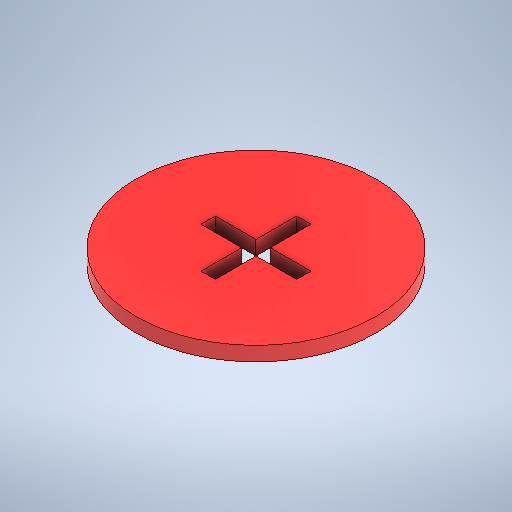
# Autodesk Inventor part: Base Arvore
Saved by Autodesk Inventor 2025 (Build 290162000, 162)
## iProperties
Created: 2024-12-03
Part Number: Base Arvore
Material: Generic
Document SubType Name: Modeling
Designer: Inteli
Density: 1 g/cm^3
Appearance: Light Red
Author: Inteli
Autodesk Inventor part; units mm, degrees
ref_plane "YZ Plane" through (0, 0, 0) normal (1, 0, 0) x (0, 1, 0)
ref_plane "XZ Plane" through (0, 0, 0) normal (0, 1, 0) x (-1, 0, 0)
ref_plane "XY Plane" through (0, 0, 0) normal (0, 0, 1) x (1, 0, 0)
sketch "Sketch1" plane through (0, 0, 0) normal (0, 1, 0) x (-1, 0, 0)
  circle A0 centre (0, 0) radius 25
  line L0 (10, 1.5) -> (-10, 1.5)
  line L1 (-10, 1.5) -> (-10, -1.5)
  line L2 (-10, -1.5) -> (10, -1.5)
  line L3 (10, -1.5) -> (10, 1.5)
  line L4 (1.5, 10) -> (-1.5, 10)
  line L5 (-1.5, 10) -> (-1.5, -10)
  line L6 (-1.5, -10) -> (1.5, -10)
  line L7 (1.5, -10) -> (1.5, 10)
  point P0 (-1.5, 1.5)
  point P1 (1.5, 1.5)
  point P2 (1.5, -1.5)
  point P3 (-1.5, -1.5)
  dimension "d0" = 50
  dimension "d1" = 20
  dimension "d2" = 3
  dimension "d3" = 1.5
  dimension "d4" = 10
  dimension "d5" = 3
  dimension "d6" = 20
  dimension "d7" = 10
  dimension "d8" = 1.5
  constraints: 16 end point, 4 parallel, 2 horizontal, 2 perpendicular, 1 centre point, 1 coincident
  measures "d0" diameter of A0
  measures "d1" distance of L2.end L1.end
  measures "d2" distance of L1.end L0.end
  measures "d3" distance from line of L2 point (0, 0)
  measures "d4" distance from line of point (0, 0) L3
  measures "d5" distance of L6.end L5.end
  measures "d6" distance of L5.end L4.end
  measures "d7" distance from line of L6 point (0, 0)
  measures "d8" distance from line of point (0, 0) L7
extrude "Extrusion1" add sketch "Sketch1" along normal blind 3
body "Solid1"
